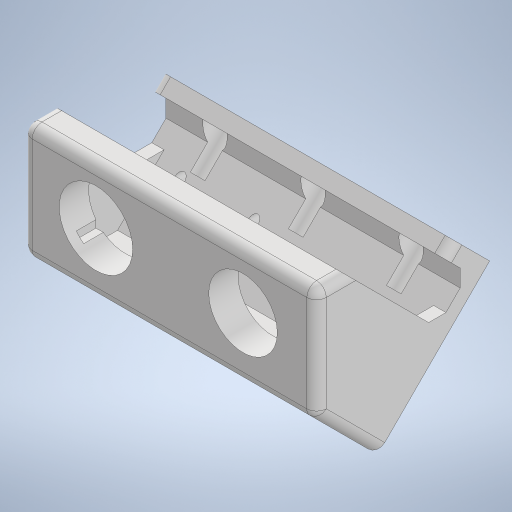
# Autodesk Inventor part: joystick_mount
Saved by Autodesk Inventor 2024.2 (Build 282272000, 272)
## iProperties
Created: 2024-06-03
Part Number: joystick_mount
Material: Generic
Document SubType Name: Modeling
Designer: Micha
Density: 1 g/cm^3
Appearance: Default
Author: Micha
Autodesk Inventor part; units mm, degrees
ref_plane "YZ Plane" through (0, 0, 0) normal (1, 0, 0) x (0, 1, 0)
ref_plane "XZ Plane" through (0, 0, 0) normal (0, 1, 0) x (-1, 0, 0)
ref_plane "XY Plane" through (0, 0, 0) normal (0, 0, 1) x (1, 0, 0)
sketch "Sketch1" plane through (0, 0, 0) normal (0, 0, 1) x (1, 0, 0)
  line L0 (0, 0) -> (110, 0)
  line L1 (110, 0) -> (110, 45)
  line L2 (110, 45) -> (0, 45)
  line L3 (0, 45) -> (0, 0)
  circle A0 centre (25, 22.5) radius 15
  circle A1 centre (85, 22.5) radius 14
  point P0 (0, 22.5)
  dimension "d0" = 45
  dimension "d1" = 30
  dimension "d4" = 25
  dimension "d5" = 28
  dimension "d6" = 60
  dimension "d7" = 110
  constraints: 8 end point, 2 centre point, 2 horizontal alignment, 2 parallel, 1 horizontal, 1 midpoint, 1 perpendicular
  measures "d0" distance of L0.end L1.end
  measures "d1" diameter of A0
  measures "d4" distance from line of L3 A0.centre
  measures "d5" diameter of A1
  measures "d6" distance of A1.centre A0.centre
  measures "d7" distance of L1.end L2.end
extrude "Extrusion1" add sketch "Sketch1" along normal blind 4
sketch "Sketch2" plane through (0, 0, 0) normal (0, 0, -1) x (-1, 0, 0)
  line L0 (-110, 45) -> (0, 45)
  line L1 (-110, 0) -> (-110, 45)
  circle A0 centre (-85, 22.5) radius 14
  line L2 (0, 0) -> (-110, 0)
  line L3 (-110, 0) -> (-110, 45)
  line L4 (0, 0) -> (-110, 0)
  line L5 (0, 45) -> (0, 0)
  line L6 (-110, 45) -> (0, 45)
  circle A1 centre (-25, 22.5) radius 15
  circle A2 centre (-85, 22.5) radius 14
  line L7 (-13, 34.5) -> (-13, 10.5)
  line L8 (-41, 10.5) -> (-41, 19.796454)
  line L9 (-41, 19.796454) -> (-41, 34.5)
  line L10 (-41, 34.5) -> (-34, 34.5)
  line L11 (-16, 34.5) -> (-13, 34.5)
  line L12 (-13, 10.5) -> (-16, 10.5)
  line L13 (-34, 10.5) -> (-41, 10.5)
  point P0 (-13, 22.5)
  point P1 (-13, 13.5)
  point P2 (-13, 31.5)
  dimension "d11" = 24
  dimension "d13" = 12
  dimension "d67" = 16
  constraints: 14 end point, 6 parallel, 4 point on circle, 3 horizontal alignment, 2 horizontal, 2 perpendicular, 1 midpoint
  measures "d11" distance of L7.start L7.end
  measures "d13" distance from line of A1.centre L7
  measures "d67" distance from line of A1.centre L9
extrude "Extrusion2" add sketch "Sketch2" along normal blind 8
sketch "Sketch3" plane through (0, 0, -8) normal (0, 0, -1) x (-1, 0, 0)
  circle A0 centre (-25, 22.5) radius 15 projected
  line L0 (-10, 7.5) -> (-40, 7.5)
  line L1 (-40, 7.5) -> (-40, 37.5)
  line L2 (-40, 37.5) -> (-10, 37.5)
  line L3 (-10, 37.5) -> (-10, 7.5)
  line L4 (-10, 7.5) -> (-40, 37.5) construction
  line L5 (-40, 7.5) -> (-10, 37.5) construction
  circle A1 centre (-40, 37.5) radius 1.65
  circle A2 centre (-10, 37.5) radius 1.65
  circle A3 centre (-40, 7.5) radius 1.65
  circle A4 centre (-10, 7.5) radius 1.65
  point P0 (0, 0)
  dimension "d16" = 30
  dimension "d17" = 30
  dimension "d18" = 3.3
  dimension "d19" = 3.3
  dimension "d20" = 3.3
  dimension "d21" = 3.3
  constraints: 12 end point, 4 centre point, 4 coincident, 2 midpoint, 2 parallel, 1 horizontal, 1 perpendicular
  measures "d16" distance of L1.end L2.end
  measures "d17" distance of L0.end L1.end
  measures "d18" diameter of A1
  measures "d19" diameter of A2
  measures "d20" diameter of A3
  measures "d21" diameter of A4
extrude "Extrusion3" cut sketch "Sketch3" against normal blind 5 contours A2 L2 L3 | L3 L2 A2 | A4 L0 L3 | L3 L0 A4 | A1 L1 L2 | L2 L1 A1 | A3 L1 L0 | L0 L1 A3
sketch "Sketch4" plane through (0, 0, 4) normal (-1, 0, 0) x (0, 0, 1)
  line L0 (-12, 0) -> (-12, 45)
  line L1 (-12, 0) -> (-31, -19)
  line L2 (-31, -19) -> (-25, -25)
  line L3 (-25, -25) -> (0, 0)
  line L4 (-12, 0) -> (0, 0)
  line L5 (-31, -19) -> (-66.355339, 16.355339)
  line L6 (-66.355339, 16.355339) -> (-62.112698, 20.59798)
  line L7 (-62.112698, 20.59798) -> (-26.757359, -14.757359)
  line L8 (-12, 0) -> (0, 0)
  line L9 (0, 45) -> (0, 0)
  line L10 (-12, 45) -> (0, 45)
  line L11 (-12, 0) -> (-12, 45)
  point P0 (-4, 0)
  dimension "d24" = 45
  dimension "d25" = 25
  dimension "d26" = 6
  dimension "d27" = 50
  constraints: 12 end point, 4 perpendicular, 1 coincident, 1 collinear, 1 point on line
  measures "d24" angle of L3 L4
  measures "d25" horizontal distance of L2.end L3.end
  measures "d26" distance of L5.end L6.end
  measures "d27" distance of L1.end L5.end
extrude "Extrusion4" add sketch "Sketch4" against normal up to surface (110 mm away) contours L4 L3 L2 L1 | L1 L5 L6 L7
sketch "Sketch5" plane through (110, 16.355339, -62.355339) normal (0, 0.7071068, -0.7071068) x (-1, 0, 0)
  line L0 (110, 0) -> (0, 0) projected
  line L1 (0, 0) -> (110, 0)
  line L2 (110, 0) -> (110, 20)
  line L3 (110, 20) -> (0, 20)
  line L4 (0, 20) -> (0, 0)
  point P0 (110, 32.526912)
  dimension "d30" = 20
  constraints: 8 end point, 2 parallel, 1 horizontal, 1 perpendicular
  measures "d30" distance of L0.start L2.end
extrude "Extrusion5" add sketch "Sketch5" along normal blind 6
sketch "Sketch7" plane through (0, 45, -8) normal (-1, 0, 0) x (0, 0, 1)
  line L0 (12, 0) -> (12, -45)
  line L1 (0, 0) -> (12, 0)
  line L2 (0, -45) -> (0, 0)
  line L3 (0, -45) -> (-14.757359, -59.757359)
  line L4 (-14.757359, -59.757359) -> (-50.112698, -24.40202)
  line L5 (-50.112698, -24.40202) -> (-40.213203, -14.502525)
  line L6 (-40.213203, -14.502525) -> (-44.455844, -10.259885)
  line L7 (-58.59798, -24.40202) -> (-44.455844, -10.259885)
  line L8 (-58.59798, -24.40202) -> (-13, -70)
  line L9 (-13, -70) -> (12, -45)
  line L10 (0, 0) -> (-37.257359, -37.257359)
  line L11 (-37.257359, -37.257359) -> (-41.5, -41.5)
  point P0 (8, -45)
  constraints: 4 end point, 2 perpendicular, 2 point on line
extrude "Extrusion7" add sketch "Sketch7" along normal blind 5
sketch "Sketch8" plane through (110, 45, 4) normal (1, 0, 0) x (0, 0, -1)
  line L0 (12, 0) -> (0, 0)
  line L1 (0, -45) -> (0, 0)
  line L2 (25, -70) -> (0, -45)
  line L3 (25, -70) -> (70.59798, -24.40202)
  line L4 (56.455844, -10.259885) -> (70.59798, -24.40202)
  line L5 (52.213203, -14.502525) -> (56.455844, -10.259885)
  line L6 (52.213203, -14.502525) -> (62.112698, -24.40202)
  line L7 (26.757359, -59.757359) -> (62.112698, -24.40202)
  line L8 (12, -45) -> (26.757359, -59.757359)
  line L9 (12, 0) -> (12, -45)
  line L10 (12, 0) -> (49.257359, -37.257359)
  point P0 (4, -45)
extrude "Extrusion8" add sketch "Sketch8" along normal blind 5
sketch "Sketch9" plane through (0, 0, -8) normal (0, 0, -1) x (-1, 0, 0)
  circle A0 centre (-40, 7.5) radius 1.65 projected
  circle A1 centre (-10, 7.5) radius 1.65 projected
  circle A2 centre (-40, 7.5) radius 2
  circle A3 centre (-10, 7.5) radius 2
  point P0 (0, 0)
  dimension "d39" = 4
  dimension "d40" = 4
  constraints: 2 centre point, 2 coincident
  measures "d39" diameter of A2
  measures "d40" diameter of A3
extrude "Extrusion9" cut sketch "Sketch9" along normal through all contours A0 | A1 | A2 | A3
sketch "Sketch10" plane through (110, 20.59798, -66.59798) normal (0, 0.7071068, -0.7071068) x (-1, 0, 0)
  circle A0 centre (15, 10) radius 2.7
  circle A1 centre (55, 10) radius 2.7
  circle A2 centre (95, 10) radius 2.7
  line L0 (-5, 20) -> (115, 20) projected
  line L1 (-5, 0) -> (-5, 20) projected
  line L2 (115, 20) -> (115, 0) projected
  line L3 (15, 10) -> (55, 10) construction
  line L4 (55, 10) -> (95, 10) construction
  point P0 (110, 32.526912)
  dimension "d43" = 5.4
  dimension "d44" = 5.4
  dimension "d45" = 5.4
  dimension "d46" = 10
  dimension "d47" = 20
  dimension "d48" = 20
  constraints: 4 end point, 3 centre point, 2 collinear, 2 horizontal alignment, 1 horizontal
  measures "d43" diameter of A0
  measures "d44" diameter of A1
  measures "d45" diameter of A2
  measures "d46" distance from line of L0 L3.start
  measures "d47" distance from line of L1 L3.start
  measures "d48" distance from line of L4.end L2
extrude "Extrusion10" cut sketch "Sketch10" against normal up to surface (6 mm away)
sketch "Sketch11" plane through (110, 16.355339, -62.355339) normal (0, -0.7071068, 0.7071068) x (1, 0, 0)
  circle A0 centre (-95, 10) radius 2.7 projected
  circle A1 centre (-95, 10) radius 2.7 projected
  circle A2 centre (-55, 10) radius 2.7 projected
  circle A3 centre (-15, 10) radius 2.7 projected
  circle A4 centre (-95, 10) radius 2.7 projected
  circle A5 centre (-95, 10) radius 5
  circle A6 centre (-55, 10) radius 5
  circle A7 centre (-15, 10) radius 5
  point P0 (-110, 32.526912)
  dimension "d51" = 10
  dimension "d52" = 10
  dimension "d53" = 10
  constraints: 3 centre point, 3 coincident
  measures "d51" diameter of A5
  measures "d52" diameter of A6
  measures "d53" diameter of A7
extrude "Extrusion11" cut sketch "Sketch11" along normal blind 15 and the other way blind 1 contours A0 | A5 | A6 | A7
fillet "Fillet1" radius 4 10 edges at (115, -12.5, -8.5) (115, 22.5, 4) (55, 0, 4) (55, 45, 4) (-5, 22.5, 4) (-5, -12.5, -8.5) (115, 45, -2) (-5, 45, -2) (115, 32.6188, -50.3345) (-5, 32.6188, -50.3345)
chamfer "Chamfer1" distance 10 angle 45 1 edges at (55, -14.7574, -22.7574)
chamfer "Chamfer2" distance 5 angle 45 6 edges at (106.5, 20.598, -58.1127) (75, 20.598, -58.1127) (35, 20.598, -58.1127) (3.5, 20.598, -58.1127) (112.5, 7.7426, -45.2574) (-2.5, 7.7426, -45.2574)
sketch "Sketch12" plane through (110, 16.355339, -62.355339) normal (0, -0.7071068, 0.7071068) x (1, 0, 0)
  circle A0 centre (-15, 10) radius 2.7 projected
  circle A1 centre (-55, 10) radius 2.7 projected
  circle A2 centre (-95, 10) radius 2.7 projected
  point P0 (-110, 32.526912)
extrude "Extrusion12" cut sketch "Sketch12" along normal through all both and the other way through all
move faces "Move1" translate (0, 0, 1.5) faces at (40.666667, 22.5, 0)
body "Solid1"
